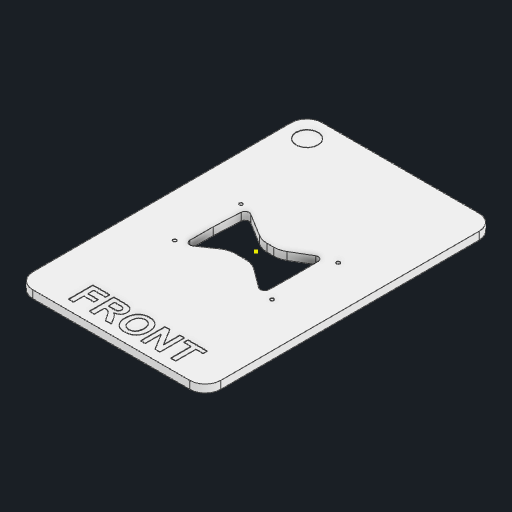
# Autodesk Inventor part: BaseBoard
Saved by Autodesk Inventor 2023 (Build 270158000, 158)
## iProperties
Created: 2022-11-10
Part Number: BaseBoard
Material: Generic
Document SubType Name: Modeling
Designer: haash
Density: 1 g/cm^3
Appearance: White
Author: haash
Autodesk Inventor part; units mm, degrees
ref_plane "YZ Plane" through (0, 0, 0) normal (1, 0, 0) x (0, 1, 0)
ref_plane "XZ Plane" through (0, 0, 0) normal (0, 1, 0) x (-1, 0, 0)
ref_plane "XY Plane" through (0, 0, 0) normal (0, 0, 1) x (1, 0, 0)
sketch "Sketch1" plane through (0, 0, 0) normal (0, 1, 0) x (-1, 0, 0)
  line L0 (-231, 355.6) -> (231, 355.6)
  line L1 (231, 355.6) -> (231, -355.6)
  line L2 (231, -355.6) -> (-231, -355.6)
  line L3 (-231, -355.6) -> (-231, 355.6)
  line L4 (-231, 355.6) -> (231, -355.6) construction
  line L5 (231, 355.6) -> (-231, -355.6) construction
  point P0 (0, 0)
  dimension "d0" = 462
  dimension "d1" = 711.2
  constraints: 12 end point, 2 midpoint, 2 parallel, 1 horizontal, 1 perpendicular
  measures "d0" distance of L0.start L0.end
  measures "d1" distance of L0.end L1.end
extrude "Extrusion1" add sketch "Sketch1" along normal blind 19.05
fillet "Fillet1" radius 38.1 4 edges at (231, 9.525, 355.6) (-231, 9.525, 355.6) (-231, 9.525, -355.6) (231, 9.525, -355.6)
sketch "Sketch2" plane through (0, 19.05, 0) normal (0, 1, 0) x (1, 0, 0)
  line L0 (152.8766, -178.8891) -> (-179.8029, -178.8891) construction
  line L1 (-179.8029, -178.8891) -> (-179.8029, 264.6836) construction
  line L2 (-179.8029, 264.6836) -> (152.8766, 264.6836) construction
  line L3 (152.8766, 264.6836) -> (152.8766, -178.8891) construction
  line L4 (0, -29.5589) -> (0, 30.9666) construction
  line L5 (0, 30.9666) -> (0, 0.7039) construction
  line L6 (97.858, 0) -> (-105.142, 0) construction
  point P0 (0, 0)
  dimension "d23" = 203
  dimension "d28" = 60.5255
  dimension "d29" = 178.8891
  dimension "d31" = 55.0186
  dimension "d32" = 152.8766
  dimension "d34" = 149.3302
  dimension "d41" = 332.6795
  constraints: 6 end point, 2 horizontal, 2 point on line, 1 midpoint, 1 vertical, 2 other
  measures "d23" distance of L6.start L6.end
  measures "d28" distance of L4.start L4.end
  measures "d29" vertical distance of L0.start L6.start
  measures "d31" distance from line of L3 L6.start
  measures "d32" distance from line of L3 L4.start
  measures "d34" distance from line of L0 L4.start
  measures "d41" distance of L0.start L0.end
sketch "Sketch3" plane through (0, 19.05, 0) normal (0, 1, 0) x (1, 0, 0)
  circle A0 centre (-177.8454, 303.3116) radius 27.0466
  point P0 (0, 0)
  constraints: 1 centre point
extrude "Extrusion2" cut sketch "Sketch3" against normal blind 1
sketch "Sketch4" plane through (0, 19.05, 0) normal (0, 1, 0) x (1, 0, 0)
  point P0 (0, 0)
sketch "Sketch5" plane through (0, 19.05, 0) normal (0, 1, 0) x (1, 0, 0)
  line L0 (-102.322, -272.8587) -> (120.5938, -272.8587) construction
  line L1 (120.5938, -272.8587) -> (120.5938, -330.1103) construction
  line L2 (120.5938, -330.1103) -> (-102.322, -330.1103) construction
  line L3 (-102.322, -330.1103) -> (-102.322, -272.8587) construction
  line L4 (-129.111, -331.4845) -> (-129.111, -271.4845)
  line L5 (-129.111, -271.4845) -> (-87.9068, -271.4845)
  line L6 (-87.9068, -271.4845) -> (-87.9068, -281.6369)
  line L7 (-87.9068, -281.6369) -> (-116.9921, -281.6369)
  line L8 (-116.9921, -281.6369) -> (-116.9921, -295.8137)
  line L9 (-116.9921, -295.8137) -> (-91.8854, -295.8137)
  line L10 (-91.8854, -295.8137) -> (-91.8854, -305.9662)
  line L11 (-91.8854, -305.9662) -> (-116.9921, -305.9662)
  line L12 (-116.9921, -305.9662) -> (-116.9921, -331.4845)
  line L13 (-116.9921, -331.4845) -> (-129.111, -331.4845)
  line L14 (-77.8915, -331.4845) -> (-77.8915, -271.4845)
  line L15 (-77.8915, -271.4845) -> (-52.3732, -271.4845)
  spline S0 degree 2 poles (-52.3732, -271.4845) (-42.7239, -271.4845) (-34.0348, -274.7314) (-28.7757, -282.9631) (-28.7757, -288.3137) knots 0 0 0 1 2 3 3 3
  spline S1 degree 2 poles (-28.7757, -288.3137) (-28.7757, -295.0363) (-36.6873, -303.8625) (-44.5989, -305.0058) knots 0 0 0 1 2 2 2
  spline S2 degree 2 poles (-44.5989, -305.0058) (-40.6659, -307.2924) (-35.544, -312.7802) (-31.1995, -319.7771) knots 0 0 0 1 2 2 2
  line L16 (-31.1995, -319.7771) -> (-23.8824, -331.4845)
  line L17 (-23.8824, -331.4845) -> (-38.3793, -331.4845)
  line L18 (-38.3793, -331.4845) -> (-47.1141, -318.4052)
  spline S3 degree 2 poles (-47.1141, -318.4052) (-51.8245, -311.4082) (-55.2543, -307.7497) (-59.0958, -306.4235) (-63.3031, -306.4235) knots 0 0 0 1 2 3 3 3
  line L19 (-63.3031, -306.4235) -> (-65.7726, -306.4235)
  line L20 (-65.7726, -306.4235) -> (-65.7726, -331.4845)
  line L21 (-65.7726, -331.4845) -> (-77.8915, -331.4845)
  line L22 (-65.7726, -296.8656) -> (-56.8092, -296.8656)
  spline S4 degree 2 poles (-56.8092, -296.8656) (-48.0745, -296.8656) (-43.73, -295.4021) (-41.2604, -291.7893) (-41.2604, -289.0912) knots 0 0 0 1 2 3 3 3
  spline S5 degree 2 poles (-41.2604, -289.0912) (-41.2604, -286.0729) (-44.5074, -282.3229) (-47.4342, -281.8198) knots 0 0 0 1 2 2 2
  spline S6 degree 2 poles (-47.4342, -281.8198) (-48.9434, -281.6369) (-56.3062, -281.6369) knots 0 0 0 1 1 1
  line L23 (-56.3062, -281.6369) -> (-65.7726, -281.6369)
  line L24 (-65.7726, -281.6369) -> (-65.7726, -296.8656)
  spline S7 degree 2 poles (-19.8123, -301.8503) (-19.8123, -292.704) (-17.0684, -286.4845) knots 0 0 0 1 1 1
  spline S8 degree 2 poles (-17.0684, -286.4845) (-15.0104, -281.9113) (-7.922, -274.5942) (-3.7147, -272.8564) knots 0 0 0 1 2 2 2
  spline S9 degree 2 poles (-3.7147, -272.8564) (1.8646, -270.4784) (9.2274, -270.4784) knots 0 0 0 1 1 1
  spline S10 degree 2 poles (9.2274, -270.4784) (22.4896, -270.4784) (38.4042, -286.9418) (38.4042, -301.5759) knots 0 0 0 1 2 2 2
  spline S11 degree 2 poles (38.4042, -301.5759) (38.4042, -316.0729) (22.581, -332.4906) (9.3646, -332.4906) knots 0 0 0 1 2 2 2
  spline S12 degree 2 poles (9.3646, -332.4906) (-3.9891, -332.4906) (-19.8123, -316.1643) (-19.8123, -301.8503) knots 0 0 0 1 2 2 2
  spline S13 degree 2 poles (-7.3275, -301.4387) (-7.3275, -311.6369) (2.0932, -322.1552) (9.3646, -322.1552) knots 0 0 0 1 2 2 2
  spline S14 degree 2 poles (9.3646, -322.1552) (16.6359, -322.1552) (25.9194, -311.7284) (25.9194, -301.3015) knots 0 0 0 1 2 2 2
  spline S15 degree 2 poles (25.9194, -301.3015) (25.9194, -290.9662) (16.8646, -280.8137) (9.3646, -280.8137) knots 0 0 0 1 2 2 2
  spline S16 degree 2 poles (9.3646, -280.8137) (1.8646, -280.8137) (-7.3275, -291.1034) (-7.3275, -301.4387) knots 0 0 0 1 2 2 2
  line L25 (47.9621, -331.4845) -> (47.9621, -271.4845)
  line L26 (47.9621, -271.4845) -> (59.7152, -271.4845)
  line L27 (59.7152, -271.4845) -> (84.3646, -311.7284)
  line L28 (84.3646, -311.7284) -> (84.3646, -271.4845)
  line L29 (84.3646, -271.4845) -> (95.5688, -271.4845)
  line L30 (95.5688, -271.4845) -> (95.5688, -331.4845)
  line L31 (95.5688, -331.4845) -> (83.4499, -331.4845)
  line L32 (83.4499, -331.4845) -> (59.1664, -292.1095)
  line L33 (59.1664, -292.1095) -> (59.1664, -331.4845)
  line L34 (59.1664, -331.4845) -> (47.9621, -331.4845)
  line L35 (121.9103, -331.4845) -> (121.9103, -281.6369)
  line L36 (121.9103, -281.6369) -> (104.1207, -281.6369)
  line L37 (104.1207, -281.6369) -> (104.1207, -271.4845)
  line L38 (104.1207, -271.4845) -> (151.7731, -271.4845)
  line L39 (151.7731, -271.4845) -> (151.7731, -281.6369)
  line L40 (151.7731, -281.6369) -> (134.0292, -281.6369)
  line L41 (134.0292, -281.6369) -> (134.0292, -331.4845)
  line L42 (134.0292, -331.4845) -> (121.9103, -331.4845)
  point P0 (0, 0)
  constraints: 2 other
extrude "Extrusion3" cut sketch "Sketch5" against normal blind 1
sketch "Sketch6" plane through (0, 19.05, 0) normal (0, 1, 0) x (1, 0, 0)
  line L0 (4.2298, -29.5589) -> (-21.0762, -29.5589)
  line L1 (12.3982, 30.9666) -> (-3.642, 30.9666)
  line L2 (82.3546, 64.3536) -> (37.925, 37.9738)
  line L3 (-29.9268, 38.433) -> (-86.7171, 73.5282)
  line L4 (-49.372, -38.3358) -> (-89.4828, -65.8681)
  line L5 (34.0297, -39.4096) -> (80.2832, -73.7401)
  line L6 (0, -29.5589) -> (0, 30.9666) construction
  line L7 (97.858, 0) -> (-105.142, 0) construction
  arc A0 (-21.0762, -29.5589) -> (-49.372, -38.3358) centre (-21.0762, -79.5589) ccw
  arc A1 (34.0297, -39.4096) -> (4.2298, -29.5589) centre (4.2298, -79.5589) ccw
  arc A2 (12.3982, 30.9666) -> (37.925, 37.9738) centre (12.3982, 80.9666) ccw
  arc A3 (-29.9268, 38.433) -> (-3.642, 30.9666) centre (-3.642, 80.9666) ccw
  arc A4 (97.4597, 55.8264) -> (82.3546, 64.3536) centre (87.4599, 55.7551) ccw
  arc A5 (80.2832, -73.7401) -> (97.0614, -65.4261) centre (86.549, -65.2981) ccw
  arc A6 (-105.142, -57.6234) -> (-89.4828, -65.8681) centre (-95.142, -57.6234) ccw
  arc A7 (-86.7171, 73.5282) -> (-101.9624, 65.5063) centre (-91.9741, 65.0214) ccw
  line L8 (-101.9624, 65.5063) -> (-105.142, 0)
  line L9 (-105.142, -57.6234) -> (-105.142, 0)
  line L10 (97.0614, -65.4261) -> (97.858, 0)
  line L11 (97.4597, 55.8264) -> (97.858, 0)
  point P0 (0, 0)
  dimension "d56" = 50
  dimension "d57" = 50
  dimension "d58" = 50
  dimension "d59" = 10
  dimension "d61" = 10
  dimension "d62" = 10
  constraints: 20 end point, 16 point on circle, 16 tangent, 8 centre point, 2 horizontal, 2 point on line, 1 equal radius, 1 vertical, 7 other
  measures "d56" radius of A0
  measures "d57" radius of A1
  measures "d58" radius of A2
  measures "d59" radius of A4
  measures "d61" radius of A6
  measures "d62" radius of A7
extrude "Extrusion4" cut sketch "Sketch6" against normal through all
sketch "Sketch7" plane through (0, 19.05, 0) normal (0, 1, 0) x (1, 0, 0)
  circle A0 centre (121.5557, -81.9528) radius 4.2334
  circle A1 centre (124.4127, 77.4269) radius 4.3443
  circle A2 centre (-119.85, 82.8926) radius 4.0735
  circle A3 centre (-124.0139, -75.9442) radius 4.2163
  point P0 (0, 0)
  constraints: 4 centre point
extrude "Extrusion5" cut sketch "Sketch7" against normal blind 1
equation "\"d57\" = d56"
equation "\"d58\" = d57"
body "Solid1"
